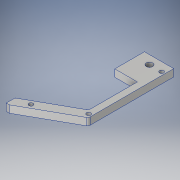
# Autodesk Inventor part: Marco_triciclo
Saved by Autodesk Inventor 2019 (Build 230136000, 136)
## iProperties
Created: 2019-11-14
Part Number: Marco_triciclo
Material: Aluminum 6061
Document SubType Name: Modeling
Designer: Domenico
Density: 2.7 g/cm^3
Appearance: Aluminum - Flat
Mass: 1547.99 g
Surface Area: 823.056 cm^2
Volume: 573.33 cm^3
altura_hoyo: 12.300 mm
Ancho_marco: 24.600 mm
d_entre_ejes: 157.401 mm
Author: Domenico
Autodesk Inventor part; units mm, degrees
ref_plane "YZ Plane" through (0, 0, 0) normal (1, 0, 0) x (0, 1, 0)
ref_plane "XZ Plane" through (0, 0, 0) normal (0, 1, 0) x (-1, 0, 0)
ref_plane "XY Plane" through (0, 0, 0) normal (0, 0, 1) x (1, 0, 0)
sketch "Sketch1" plane through (0, 0, 0) normal (0, 1, 0) x (-1, 0, 0)
  line L0 (0, 0) -> (108.6, 0)
  line L1 (108.6, 0) -> (108.6, -110.4)
  line L2 (108.6, -110.4) -> (0, -110.4)
  line L3 (0, -110.4) -> (0, 0)
  circle A0 centre (12.3, -77.7) radius 7.8
  circle A1 centre (57.3, -77.7) radius 12
  dimension "d0" = 108.6
  dimension "d1" = 110.4
  dimension "d2" = 15.6
  dimension "altura_hoyo" = 12.3
  dimension "d5" = 32.7
  dimension "d6" = 24
  dimension "d7" = 45
  constraints: 8 end point, 2 centre point, 2 parallel, 1 horizontal, 1 horizontal alignment, 1 perpendicular
  measures "d0" distance of L1.end L2.end
  measures "d1" distance between parallel lines of L2 L0
  measures "d2" diameter of A0
  measures "altura_hoyo" distance from line of L3 A0.centre
  measures "d5" distance from line of L2 A0.centre
  measures "d6" diameter of A1
  measures "d7" distance of A0.centre A1.centre
extrude "Extrusion1" add sketch "Sketch1" along normal blind 27
sketch "Sketch2" plane through (0, 27, 0) normal (0, 1, 0) x (1, 0, 0)
  line L0 (0, 110.4) -> (-108.6, 110.4) construction
  line L1 (0, 0) -> (0, -193.5)
  line L2 (0, -193.5) -> (0, -206.2)
  line L3 (0, -206.2) -> (-188.5967, -311.4961)
  line L4 (-24.6, 0) -> (-24.6, -180.8)
  line L5 (-188.5967, -272.3616) -> (-24.6, -180.8)
  line L6 (-188.5967, -311.4961) -> (-188.5967, -272.3616)
  circle A0 centre (-12.3, -193.5) radius 7.8
  circle A1 centre (-12.3, 77.7) radius 7.8 construction
  line L7 (-108.6, 0) -> (0, 0) projected
  line L8 (0, 0) -> (-24.6, 0)
  line L9 (-12.3, -193.5) -> (-149.732, -270.2302) construction
  line L10 (0, -206.2) -> (-12.3, -193.5) construction
  line L11 (-31.4236, -173.7545) -> (-12.3, -193.5) construction
  circle A2 centre (-149.732, -270.2302) radius 7.8
  dimension "d10" = 303.9
  dimension "d11" = 12.7
  dimension "d12" = 119.175
  dimension "Ancho_marco" = 24.6
  dimension "d18" = 15.6
  dimension "d21" = 216
  dimension "d26" = 12.3
  dimension "d_entre_ejes" = 157.401
  dimension "d28" = 15.6
  dimension "d31" = 193.5
  constraints: 20 end point, 4 vertical, 2 centre point, 2 parallel, 2 point on line, 1 coincident, 1 collinear, 1 horizontal alignment
  measures "d10" distance from line of L0 L1.end
  measures "d11" distance of L1.end L2.end
  measures "d12" angle of L1 L3
  measures "Ancho_marco" distance between parallel lines of L1 L4
  measures "d18" diameter of A0
  measures "d21" distance of L2.end L3.end
  measures "d26" horizontal distance of L4.end L9.start
  measures "d_entre_ejes" distance of L9.start L9.end
  measures "d28" diameter of A2
  measures "d31" distance of L1.start L1.end
extrude "Extrusion2" add sketch "Sketch2" against normal blind 27 contours L1 L2 L3 L6 L5 L4 L7 | A2
fillet "Fillet1" radius 10 2 edges at (-24.6, 13.5, 180.8) (0, 13.5, 206.2)
sketch "Sketch3" plane through (0, 27, 0) normal (0, 1, 0) x (1, 0, 0)
  line L0 (-188.5967, -272.3616) -> (-188.5967, -311.4961) projected
  line L1 (-188.5967, -311.4961) -> (-200.2967, -311.4961)
  line L2 (-200.2967, -311.4961) -> (-200.2967, -278.8939)
  line L3 (-188.5967, -311.4961) -> (-188.5967, -272.3616) projected
  line L4 (-188.5967, -272.3616) -> (-200.2967, -278.8939)
  line L5 (-29.7252, -183.6615) -> (-188.5967, -272.3616) projected
  point P0 (0, 0)
  dimension "d23" = 11.7
  constraints: 6 end point, 1 collinear, 1 horizontal, 1 perpendicular
  measures "d23" distance of L0.end L1.end
extrude "Extrusion3" add sketch "Sketch3" against normal blind 27
extrude "Extrusion4" cut sketch "Sketch2" against normal blind 27 contours A2
equation "\"d2\" = d18"
equation "\"d11\" = 0.5 * D_eje"
equation "\"d18\" = d28"
equation "\"D_eje\" = 25.4"
body "Solid1"
